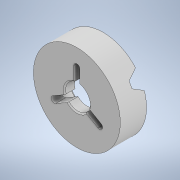
# Autodesk Inventor part: encoder_ma_holder_1
Saved by Autodesk Inventor 2020 (Build 240168000, 168)
## iProperties
Created: 2020-10-12
Part Number: encoder_ma_holder_1
Material: Generic
Document SubType Name: Modeling
Designer: Shuang Peng
Density: 1 g/cm^3
Appearance: Default
Author: Shuang Peng
Autodesk Inventor part; units mm, degrees
ref_plane "YZ Plane" through (0, 0, 0) normal (1, 0, 0) x (0, 1, 0)
ref_plane "XZ Plane" through (0, 0, 0) normal (0, 1, 0) x (-1, 0, 0)
ref_plane "XY Plane" through (0, 0, 0) normal (0, 0, 1) x (1, 0, 0)
sketch "Sketch1" plane through (0, 0, 0) normal (0, 0, 1) x (1, 0, 0)
  circle A0 centre (0, 0) radius 9
  circle A1 centre (0, 0) radius 10.75
  dimension "d0" = 18
  dimension "d1" = 21.5
  constraints: 2 centre point, 2 coincident
  measures "d0" diameter of A0
  measures "d1" diameter of A1
extrude "Extrusion1" add sketch "Sketch1" against normal blind 4
sketch "Sketch2" plane through (0, 0, 0) normal (0, 0, 1) x (1, 0, 0)
  circle A0 centre (0, 0) radius 10.75 projected
  circle A1 centre (0, 0) radius 3
  dimension "d4" = 6
  constraints: 1 centre point, 1 coincident
  measures "d4" diameter of A1
extrude "Extrusion2" add sketch "Sketch2" along normal blind 2.5
sketch "Sketch3" plane through (0, 0, 2.5) normal (0, 0, 1) x (1, 0, 0)
  line L0 (0, -6.5) -> (0, 6.5) construction
  line L1 (0.75, -6.5) -> (0.75, 6.5)
  line L2 (-0.75, 6.5) -> (-0.75, -6.5)
  arc A0 (-0.75, -6.5) -> (0.75, -6.5) centre (0, -6.5) ccw
  arc A1 (0.75, 6.5) -> (-0.75, 6.5) centre (0, 6.5) ccw
  circle A2 centre (0, 0) radius 10.75 projected
  circle A3 centre (0, 0) radius 3 projected
  point P0 (-0.75, 2.9047)
  point P1 (0.75, 2.9047)
  dimension "d7" = 6.5
  dimension "d8" = 1.5
  constraints: 8 end point, 4 point on circle, 4 tangent, 2 centre point, 1 midpoint, 1 parallel, 1 vertical
  measures "d7" distance of point (0, 0) L0.end
  measures "d8" diameter of A1
extrude "Extrusion3" cut sketch "Sketch3" against normal blind 2.5 contours A3 L2 A1 L1
pattern_circular "Circular Pattern1" count 3 over 360 about axis through (0, 0, 0) along (0, 0, 1) of "Extrusion3"
ref_plane "Work Plane1" through (0, 0, -1.5) normal (0, 0, -1) x (-1, 0, 0)
sketch "Sketch4" plane through (0, 0, -1.5) normal (0, 0, -1) x (-1, 0, 0)
  line L0 (-6.0042, -2.6005) -> (-2.8906, -0.8028) projected
  arc A0 (-0.75, 2.9047) -> (-2.8906, -0.8028) centre (0, 0) ccw projected
  line L1 (-0.75, 2.9047) -> (-0.75, 6.5) projected
  arc A1 (0.75, 6.5) -> (-0.75, 6.5) centre (0, 6.5) ccw projected
  line L2 (0.75, 6.5) -> (0.75, 2.9047) projected
  arc A2 (2.8906, -0.8028) -> (0.75, 2.9047) centre (0, 0) ccw projected
  line L3 (2.8906, -0.8028) -> (6.0042, -2.6005) projected
  arc A3 (5.2542, -3.8995) -> (6.0042, -2.6005) centre (5.6292, -3.25) ccw projected
  line L4 (5.2542, -3.8995) -> (2.1406, -2.1019) projected
  arc A4 (-2.1406, -2.1019) -> (2.1406, -2.1019) centre (0, 0) ccw projected
  line L5 (-2.1406, -2.1019) -> (-5.2542, -3.8995) projected
  arc A5 (-6.0042, -2.6005) -> (-5.2542, -3.8995) centre (-5.6292, -3.25) ccw projected
  circle A6 centre (0, 0) radius 9 projected
  line L6 (0, 0) -> (-5.6292, -3.25)
  line L7 (17.3205, 10) -> (-17.3205, -10) construction
  line L8 (16.9455, 10.6495) -> (-17.6955, -9.3505)
  line L9 (-16.9455, -10.6495) -> (17.6955, 9.3505)
  arc A7 (17.6955, 9.3505) -> (16.9455, 10.6495) centre (17.3205, 10) ccw
  arc A8 (-17.6955, -9.3505) -> (-16.9455, -10.6495) centre (-17.3205, -10) ccw
  circle A9 centre (0, 0) radius 10.75 projected
  circle A10 centre (0, 0) radius 9 projected
  point P0 (9.6621, 4.7124)
  point P1 (8.9121, 6.0114)
  point P2 (7.3921, 5.1339)
  point P3 (8.1421, 3.8348)
  dimension "d15" = 20
  dimension "d16" = 1.5
  constraints: 10 end point, 4 point on circle, 4 tangent, 2 centre point, 2 parallel, 1 midpoint
  measures "d15" distance of L6.start L7.end
  measures "d16" diameter of A8
extrude "Extrusion4" cut sketch "Sketch4" along normal blind 2.5 contours L8 A9 L9 A6 picked at (8.5735, 4.2763)
pattern_circular "Circular Pattern2" count 3 over 360 about axis through (0, 0, 0) along (0, 0, -1) of "Extrusion4"
chamfer "Chamfer1" distance 2.5 angle 30 1 edges at (-8.9021, 4.2736, -4) measured on face at (-8.9021, 4.2736, -3.5)
chamfer "Chamfer2" distance 2.5 angle 30 1 edges at (-8.1521, 5.5726, -4) measured on face at (-8.1521, 5.5726, -3.5)
chamfer "Chamfer3" distance 2.5 angle 30 1 edges at (-0.75, -9.8463, -4) measured on face at (-0.75, -9.8463, -3.5)
chamfer "Chamfer4" distance 2.5 angle 30 1 edges at (0.75, -9.8463, -4) measured on face at (0.75, -9.8463, -3.5)
chamfer "Chamfer5" distance 2.5 angle 30 1 edges at (8.9021, 4.2736, -4) measured on face at (8.9021, 4.2736, -3.5)
chamfer "Chamfer6" distance 2.5 angle 30 1 edges at (8.1521, 5.5726, -4) measured on face at (8.1521, 5.5726, -3.5)
chamfer "Chamfer7" distance 0.5 angle 45 4 edges at (-7.7942, -4.5, -4) (8.9136, 1.2444, -4) (7.0972, -5.5345, -4) (0, 9, -4)
thicken "Thicken1" operation add thickness 0.07 both sides no extend neighbours yes toward (0.8464931, 0.5323997, 0) faces at (2.5395, 1.5972, 1.6667)
thicken "Thicken2" operation add thickness 0.07 both sides no extend neighbours yes toward (0.6585189, -0.7525642, 0) faces at (1.9756, -2.2577, 1.6667)
thicken "Thicken3" operation add thickness 0.07 both sides no extend neighbours yes toward (-0.3224803, 0.9465762, 0) faces at (-0.9674, 2.8397, 0.8333)
chamfer "Chamfer8" distance 0.3 angle 45 3 edges at (2.6587, 1.535, 2.5) (0, -3.07, 2.5) (-2.6587, 1.535, 2.5)
thicken "Thicken4" operation add thickness 0.02 both sides no extend neighbours yes toward (0.6438873, 0.7651203, 0) faces at (5.795, 6.8861, -2.0016)
body "Solid1"
